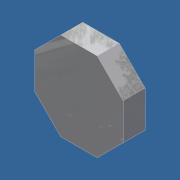
# Autodesk Inventor part: Oktagon
Saved by Autodesk Inventor 2018.2 (Build 222227000, 227)
## iProperties
Created: 2018-10-01
Part Number: Oktagon
Material: Kst - PVC (rigid/white)
Document SubType Name: Modeling
Designer: N.Grubert
Density: 1.38 g/cm^3
Appearance: Glatt - weiß
Fläche: 0 cm²
Gewicht: 0 g
Material: geeigneten Werkstoff auswählen !
Dateiname: P:\INVENTOR\Inventor 2018\Templates\ILT\Norm.ipt
Bez_eng: bolt
Bez_french: boulon
Author: N.Grubert
Autodesk Inventor part; units mm, degrees
ref_plane "YZ Plane" through (0, 0, 0) normal (1, 0, 0) x (0, 1, 0)
ref_plane "XZ Plane" through (0, 0, 0) normal (0, 1, 0) x (-1, 0, 0)
ref_plane "XY Plane" through (0, 0, 0) normal (0, 0, 1) x (1, 0, 0)
sketch "Skizze4" plane through (0, 0, 0) normal (0, 1, 0) x (-1, 0, 0)
  line L0 (77, 0) -> (-77, 0) construction
  line L1 (0, -77) -> (0, 77) construction
  line L2 (27, 37.5) -> (-27, 37.5) construction
  line L3 (-27, 37.5) -> (-27, -37.5) construction
  line L4 (-27, -37.5) -> (27, -37.5) construction
  line L5 (27, -37.5) -> (27, 37.5) construction
  line L6 (55, -22.7817) -> (22.7817, -55)
  line L7 (22.7817, -55) -> (-22.7817, -55)
  line L8 (-22.7817, -55) -> (-55, -22.7817)
  line L9 (-55, -22.7817) -> (-55, 22.7817)
  line L10 (-55, 22.7817) -> (-22.7817, 55)
  line L11 (-22.7817, 55) -> (22.7817, 55)
  line L12 (22.7817, 55) -> (55, 22.7817)
  line L13 (55, 22.7817) -> (55, -22.7817)
  line L14 (52.5, -21.7462) -> (21.7462, -52.5)
  line L15 (21.7462, -52.5) -> (-21.7462, -52.5)
  line L16 (-21.7462, -52.5) -> (-52.5, -21.7462)
  line L17 (-52.5, -21.7462) -> (-52.5, 21.7462)
  line L18 (-52.5, 21.7462) -> (-21.7462, 52.5)
  line L19 (-21.7462, 52.5) -> (21.7462, 52.5)
  line L20 (21.7462, 52.5) -> (52.5, 21.7462)
  line L21 (52.5, 21.7462) -> (52.5, -21.7462)
  point P0 (0, 0)
  point P1 (0, 0)
  dimension "d4" = 75
  dimension "d5" = 54
  dimension "d7" = 2.5
  dimension "d12" = 105
  constraints: 40 end point, 2 parallel, 1 coincident, 1 horizontal, 1 perpendicular, 27 other
  measures "d4" distance between parallel lines of L4 L2
  measures "d5" distance between parallel lines of L3 L5
  measures "d7" distance between parallel lines of L13 L21
  measures "d12" distance between parallel lines of L17 L21
extrude "Extrusion2" add sketch "Skizze4" along normal blind 25
sketch "Skizze5" plane through (0, 0, 0) normal (0, -1, 0) x (1, 0, 0)
  line L0 (21.7462, -52.5) -> (-21.7462, -52.5) projected
  line L1 (-21.7462, -52.5) -> (-52.5, -21.7462) projected
  line L2 (-52.5, -21.7462) -> (-52.5, 21.7462) projected
  line L3 (-52.5, 21.7462) -> (-21.7462, 52.5) projected
  line L4 (-21.7462, 52.5) -> (21.7462, 52.5) projected
  line L5 (21.7462, 52.5) -> (52.5, 21.7462) projected
  line L6 (52.5, 21.7462) -> (52.5, -21.7462) projected
  line L7 (52.5, -21.7462) -> (21.7462, -52.5) projected
  line L8 (-55, -22.7817) -> (-22.7817, -55) projected
  line L9 (-22.7817, -55) -> (22.7817, -55) projected
  line L10 (22.7817, -55) -> (55, -22.7817) projected
  line L11 (55, -22.7817) -> (55, 22.7817) projected
  line L12 (55, 22.7817) -> (22.7817, 55) projected
  line L13 (22.7817, 55) -> (-22.7817, 55) projected
  line L14 (-22.7817, 55) -> (-55, 22.7817) projected
  line L15 (-55, 22.7817) -> (-55, -22.7817) projected
  point P0 (0, 0)
extrude "Extrusion3" add sketch "Skizze5" along normal blind 2.5 contours L0 L1 L2 L3 L4 L5 L6 L7 | L15 L14 L13 L12 L11 L10 L9 L8
